Autodesk Fusion 360 part; units mm, degrees
(part 2 of 2)
sketch "Sketch4" plane through (0, 0, 8) normal (0, 0, 1) x (-1, 0, 0)
  line L0 (-123.1754, -6.5) -> (-116.8246, -6.5)
  line L1 (-116.8246, -6.5) -> (-113.6491, -12)
  line L2 (-113.6491, -12) -> (-116.8246, -17.5)
  line L3 (-116.8246, -17.5) -> (-123.1754, -17.5)
  line L4 (-123.1754, -17.5) -> (-126.3509, -12)
  line L5 (-126.3509, -12) -> (-123.1754, -6.5)
  line L6 (-39.1754, -6.5) -> (-32.8246, -6.5)
  line L7 (-32.8246, -6.5) -> (-29.6491, -12)
  line L8 (-29.6491, -12) -> (-32.8246, -17.5)
  line L9 (-32.8246, -17.5) -> (-39.1754, -17.5)
  line L10 (-39.1754, -17.5) -> (-42.3509, -12)
  line L11 (-42.3509, -12) -> (-39.1754, -6.5)
  line L12 (-123.1754, -28.5) -> (-116.8246, -28.5)
  line L13 (-116.8246, -28.5) -> (-113.6491, -34)
  line L14 (-113.6491, -34) -> (-116.8246, -39.5)
  line L15 (-116.8246, -39.5) -> (-123.1754, -39.5)
  line L16 (-123.1754, -39.5) -> (-126.3509, -34)
  line L17 (-126.3509, -34) -> (-123.1754, -28.5)
  line L18 (-39.1754, -28.5) -> (-32.8246, -28.5)
  line L19 (-32.8246, -28.5) -> (-29.6491, -34)
  line L20 (-29.6491, -34) -> (-32.8246, -39.5)
  line L21 (-32.8246, -39.5) -> (-39.1754, -39.5)
  line L22 (-39.1754, -39.5) -> (-42.3509, -34)
  line L23 (-42.3509, -34) -> (-39.1754, -28.5)
  line L24 (-123.1754, -50.5) -> (-116.8246, -50.5)
  line L25 (-116.8246, -50.5) -> (-113.6491, -56)
  line L26 (-113.6491, -56) -> (-116.8246, -61.5)
  line L27 (-116.8246, -61.5) -> (-123.1754, -61.5)
  line L28 (-123.1754, -61.5) -> (-126.3509, -56)
  line L29 (-126.3509, -56) -> (-123.1754, -50.5)
  line L30 (-39.1754, -50.5) -> (-32.8246, -50.5)
  line L31 (-32.8246, -50.5) -> (-29.6491, -56)
  line L32 (-29.6491, -56) -> (-32.8246, -61.5)
  line L33 (-32.8246, -61.5) -> (-39.1754, -61.5)
  line L34 (-39.1754, -61.5) -> (-42.3509, -56)
  line L35 (-42.3509, -56) -> (-39.1754, -50.5)
  line L36 (-123.1754, -72.5) -> (-116.8246, -72.5)
  line L37 (-116.8246, -72.5) -> (-113.6491, -78)
  line L38 (-113.6491, -78) -> (-116.8246, -83.5)
  line L39 (-116.8246, -83.5) -> (-123.1754, -83.5)
  line L40 (-123.1754, -83.5) -> (-126.3509, -78)
  line L41 (-126.3509, -78) -> (-123.1754, -72.5)
  line L42 (-39.1754, -72.5) -> (-32.8246, -72.5)
  line L43 (-32.8246, -72.5) -> (-29.6491, -78)
  line L44 (-29.6491, -78) -> (-32.8246, -83.5)
  line L45 (-32.8246, -83.5) -> (-39.1754, -83.5)
  line L46 (-39.1754, -83.5) -> (-42.3509, -78)
  line L47 (-42.3509, -78) -> (-39.1754, -72.5)
  line L48 (-123.1754, -94.5) -> (-116.8246, -94.5)
  line L49 (-116.8246, -94.5) -> (-113.6491, -100)
  line L50 (-113.6491, -100) -> (-116.8246, -105.5)
  line L51 (-116.8246, -105.5) -> (-123.1754, -105.5)
  line L52 (-123.1754, -105.5) -> (-126.3509, -100)
  line L53 (-126.3509, -100) -> (-123.1754, -94.5)
  line L54 (-39.1754, -94.5) -> (-32.8246, -94.5)
  line L55 (-32.8246, -94.5) -> (-29.6491, -100)
  line L56 (-29.6491, -100) -> (-32.8246, -105.5)
  line L57 (-32.8246, -105.5) -> (-39.1754, -105.5)
  line L58 (-39.1754, -105.5) -> (-42.3509, -100)
  line L59 (-42.3509, -100) -> (-39.1754, -94.5)
  line L60 (-123.1754, -116.5) -> (-116.8246, -116.5)
  line L61 (-116.8246, -116.5) -> (-113.6491, -122)
  line L62 (-113.6491, -122) -> (-116.8246, -127.5)
  line L63 (-116.8246, -127.5) -> (-123.1754, -127.5)
  line L64 (-123.1754, -127.5) -> (-126.3509, -122)
  line L65 (-126.3509, -122) -> (-123.1754, -116.5)
  line L66 (-18.1754, -127.5) -> (-21.3509, -122)
  line L67 (-21.3509, -122) -> (-18.1754, -116.5)
  line L68 (-18.1754, -116.5) -> (-11.8246, -116.5)
  line L69 (-11.8246, -116.5) -> (-8.6491, -122)
  line L70 (-8.6491, -122) -> (-11.8246, -127.5)
  line L71 (-11.8246, -127.5) -> (-18.1754, -127.5)
  line L72 (-60.1754, -116.5) -> (-53.8246, -116.5)
  line L73 (-53.8246, -116.5) -> (-50.6491, -122)
  line L74 (-50.6491, -122) -> (-53.8246, -127.5)
  line L75 (-53.8246, -127.5) -> (-60.1754, -127.5)
  line L76 (-60.1754, -127.5) -> (-63.3509, -122)
  line L77 (-63.3509, -122) -> (-60.1754, -116.5)
  line L78 (-144.1754, -116.5) -> (-137.8246, -116.5)
  line L79 (-137.8246, -116.5) -> (-134.6491, -122)
  line L80 (-134.6491, -122) -> (-137.8246, -127.5)
  line L81 (-137.8246, -127.5) -> (-144.1754, -127.5)
  line L82 (-144.1754, -127.5) -> (-147.3509, -122)
  line L83 (-147.3509, -122) -> (-144.1754, -116.5)
  line L84 (-60.1754, -94.5) -> (-53.8246, -94.5)
  line L85 (-53.8246, -94.5) -> (-50.6491, -100)
  line L86 (-50.6491, -100) -> (-53.8246, -105.5)
  line L87 (-53.8246, -105.5) -> (-60.1754, -105.5)
  line L88 (-60.1754, -105.5) -> (-63.3509, -100)
  line L89 (-63.3509, -100) -> (-60.1754, -94.5)
  line L90 (-144.1754, -94.5) -> (-137.8246, -94.5)
  line L91 (-137.8246, -94.5) -> (-134.6491, -100)
  line L92 (-134.6491, -100) -> (-137.8246, -105.5)
  line L93 (-137.8246, -105.5) -> (-144.1754, -105.5)
  line L94 (-144.1754, -105.5) -> (-147.3509, -100)
  line L95 (-147.3509, -100) -> (-144.1754, -94.5)
  line L96 (-60.1754, -72.5) -> (-53.8246, -72.5)
  line L97 (-53.8246, -72.5) -> (-50.6491, -78)
  line L98 (-50.6491, -78) -> (-53.8246, -83.5)
  line L99 (-53.8246, -83.5) -> (-60.1754, -83.5)
  line L100 (-60.1754, -83.5) -> (-63.3509, -78)
  line L101 (-63.3509, -78) -> (-60.1754, -72.5)
  line L102 (-144.1754, -72.5) -> (-137.8246, -72.5)
  line L103 (-137.8246, -72.5) -> (-134.6491, -78)
  line L104 (-134.6491, -78) -> (-137.8246, -83.5)
  line L105 (-137.8246, -83.5) -> (-144.1754, -83.5)
  line L106 (-144.1754, -83.5) -> (-147.3509, -78)
  line L107 (-147.3509, -78) -> (-144.1754, -72.5)
  line L108 (-60.1754, -50.5) -> (-53.8246, -50.5)
  line L109 (-53.8246, -50.5) -> (-50.6491, -56)
  line L110 (-50.6491, -56) -> (-53.8246, -61.5)
  line L111 (-53.8246, -61.5) -> (-60.1754, -61.5)
  line L112 (-60.1754, -61.5) -> (-63.3509, -56)
  line L113 (-63.3509, -56) -> (-60.1754, -50.5)
  line L114 (-144.1754, -50.5) -> (-137.8246, -50.5)
  line L115 (-137.8246, -50.5) -> (-134.6491, -56)
  line L116 (-134.6491, -56) -> (-137.8246, -61.5)
  line L117 (-137.8246, -61.5) -> (-144.1754, -61.5)
  line L118 (-144.1754, -61.5) -> (-147.3509, -56)
  line L119 (-147.3509, -56) -> (-144.1754, -50.5)
  line L120 (-60.1754, -28.5) -> (-53.8246, -28.5)
  line L121 (-53.8246, -28.5) -> (-50.6491, -34)
  line L122 (-50.6491, -34) -> (-53.8246, -39.5)
  line L123 (-53.8246, -39.5) -> (-60.1754, -39.5)
  line L124 (-60.1754, -39.5) -> (-63.3509, -34)
  line L125 (-63.3509, -34) -> (-60.1754, -28.5)
  line L126 (-144.1754, -28.5) -> (-137.8246, -28.5)
  line L127 (-137.8246, -28.5) -> (-134.6491, -34)
  line L128 (-134.6491, -34) -> (-137.8246, -39.5)
  line L129 (-137.8246, -39.5) -> (-144.1754, -39.5)
  line L130 (-144.1754, -39.5) -> (-147.3509, -34)
  line L131 (-147.3509, -34) -> (-144.1754, -28.5)
  line L132 (-60.1754, -6.5) -> (-53.8246, -6.5)
  line L133 (-53.8246, -6.5) -> (-50.6491, -12)
  line L134 (-50.6491, -12) -> (-53.8246, -17.5)
  line L135 (-53.8246, -17.5) -> (-60.1754, -17.5)
  line L136 (-60.1754, -17.5) -> (-63.3509, -12)
  line L137 (-63.3509, -12) -> (-60.1754, -6.5)
  line L138 (-144.1754, -6.5) -> (-137.8246, -6.5)
  line L139 (-137.8246, -6.5) -> (-134.6491, -12)
  line L140 (-134.6491, -12) -> (-137.8246, -17.5)
  line L141 (-137.8246, -17.5) -> (-144.1754, -17.5)
  line L142 (-144.1754, -17.5) -> (-147.3509, -12)
  line L143 (-147.3509, -12) -> (-144.1754, -6.5)
  line L144 (-102.1754, -6.5) -> (-95.8246, -6.5)
  line L145 (-95.8246, -6.5) -> (-92.6491, -12)
  line L146 (-92.6491, -12) -> (-95.8246, -17.5)
  line L147 (-95.8246, -17.5) -> (-102.1754, -17.5)
  line L148 (-102.1754, -17.5) -> (-105.3509, -12)
  line L149 (-105.3509, -12) -> (-102.1754, -6.5)
  line L150 (-18.1754, -6.5) -> (-11.8246, -6.5)
  line L151 (-11.8246, -6.5) -> (-8.6491, -12)
  line L152 (-8.6491, -12) -> (-11.8246, -17.5)
  line L153 (-11.8246, -17.5) -> (-18.1754, -17.5)
  line L154 (-18.1754, -17.5) -> (-21.3509, -12)
  line L155 (-21.3509, -12) -> (-18.1754, -6.5)
  line L156 (-102.1754, -28.5) -> (-95.8246, -28.5)
  line L157 (-95.8246, -28.5) -> (-92.6491, -34)
  line L158 (-92.6491, -34) -> (-95.8246, -39.5)
  line L159 (-95.8246, -39.5) -> (-102.1754, -39.5)
  line L160 (-102.1754, -39.5) -> (-105.3509, -34)
  line L161 (-105.3509, -34) -> (-102.1754, -28.5)
  line L162 (-18.1754, -28.5) -> (-11.8246, -28.5)
  line L163 (-11.8246, -28.5) -> (-8.6491, -34)
  line L164 (-8.6491, -34) -> (-11.8246, -39.5)
  line L165 (-11.8246, -39.5) -> (-18.1754, -39.5)
  line L166 (-18.1754, -39.5) -> (-21.3509, -34)
  line L167 (-21.3509, -34) -> (-18.1754, -28.5)
  line L168 (-102.1754, -50.5) -> (-95.8246, -50.5)
  line L169 (-95.8246, -50.5) -> (-92.6491, -56)
  line L170 (-92.6491, -56) -> (-95.8246, -61.5)
  line L171 (-95.8246, -61.5) -> (-102.1754, -61.5)
  line L172 (-102.1754, -61.5) -> (-105.3509, -56)
  line L173 (-105.3509, -56) -> (-102.1754, -50.5)
  line L174 (-18.1754, -50.5) -> (-11.8246, -50.5)
  line L175 (-11.8246, -50.5) -> (-8.6491, -56)
  line L176 (-8.6491, -56) -> (-11.8246, -61.5)
  line L177 (-11.8246, -61.5) -> (-18.1754, -61.5)
  line L178 (-18.1754, -61.5) -> (-21.3509, -56)
  line L179 (-21.3509, -56) -> (-18.1754, -50.5)
  line L180 (-102.1754, -72.5) -> (-95.8246, -72.5)
  line L181 (-95.8246, -72.5) -> (-92.6491, -78)
  line L182 (-92.6491, -78) -> (-95.8246, -83.5)
  line L183 (-95.8246, -83.5) -> (-102.1754, -83.5)
  line L184 (-102.1754, -83.5) -> (-105.3509, -78)
  line L185 (-105.3509, -78) -> (-102.1754, -72.5)
  line L186 (-18.1754, -72.5) -> (-11.8246, -72.5)
  line L187 (-11.8246, -72.5) -> (-8.6491, -78)
  line L188 (-8.6491, -78) -> (-11.8246, -83.5)
  line L189 (-11.8246, -83.5) -> (-18.1754, -83.5)
  line L190 (-18.1754, -83.5) -> (-21.3509, -78)
  line L191 (-21.3509, -78) -> (-18.1754, -72.5)
  line L192 (-102.1754, -94.5) -> (-95.8246, -94.5)
  line L193 (-95.8246, -94.5) -> (-92.6491, -100)
  line L194 (-92.6491, -100) -> (-95.8246, -105.5)
  line L195 (-95.8246, -105.5) -> (-102.1754, -105.5)
  line L196 (-102.1754, -105.5) -> (-105.3509, -100)
  line L197 (-105.3509, -100) -> (-102.1754, -94.5)
  line L198 (-18.1754, -94.5) -> (-11.8246, -94.5)
  line L199 (-11.8246, -94.5) -> (-8.6491, -100)
  line L200 (-8.6491, -100) -> (-11.8246, -105.5)
  line L201 (-11.8246, -105.5) -> (-18.1754, -105.5)
  line L202 (-18.1754, -105.5) -> (-21.3509, -100)
  line L203 (-21.3509, -100) -> (-18.1754, -94.5)
  line L204 (-102.1754, -116.5) -> (-95.8246, -116.5)
  line L205 (-95.8246, -116.5) -> (-92.6491, -122)
  line L206 (-92.6491, -122) -> (-95.8246, -127.5)
  line L207 (-95.8246, -127.5) -> (-102.1754, -127.5)
  line L208 (-102.1754, -127.5) -> (-105.3509, -122)
  line L209 (-105.3509, -122) -> (-102.1754, -116.5)
  line L210 (-39.1754, -116.5) -> (-32.8246, -116.5)
  line L211 (-32.8246, -116.5) -> (-29.6491, -122)
  line L212 (-29.6491, -122) -> (-32.8246, -127.5)
  line L213 (-32.8246, -127.5) -> (-39.1754, -127.5)
  line L214 (-39.1754, -127.5) -> (-42.3509, -122)
  line L215 (-42.3509, -122) -> (-39.1754, -116.5)
  line L216 (-81.1754, -116.5) -> (-74.8246, -116.5)
  line L217 (-74.8246, -116.5) -> (-71.6491, -122)
  line L218 (-71.6491, -122) -> (-74.8246, -127.5)
  line L219 (-74.8246, -127.5) -> (-81.1754, -127.5)
  line L220 (-81.1754, -127.5) -> (-84.3509, -122)
  line L221 (-84.3509, -122) -> (-81.1754, -116.5)
  line L222 (-165.1754, -116.5) -> (-158.8246, -116.5)
  line L223 (-158.8246, -116.5) -> (-155.6491, -122)
  line L224 (-155.6491, -122) -> (-158.8246, -127.5)
  line L225 (-158.8246, -127.5) -> (-165.1754, -127.5)
  line L226 (-165.1754, -127.5) -> (-168.3509, -122)
  line L227 (-168.3509, -122) -> (-165.1754, -116.5)
  line L228 (-81.1754, -94.5) -> (-74.8246, -94.5)
  line L229 (-74.8246, -94.5) -> (-71.6491, -100)
  line L230 (-71.6491, -100) -> (-74.8246, -105.5)
  line L231 (-74.8246, -105.5) -> (-81.1754, -105.5)
  line L232 (-81.1754, -105.5) -> (-84.3509, -100)
  line L233 (-84.3509, -100) -> (-81.1754, -94.5)
  line L234 (-165.1754, -94.5) -> (-158.8246, -94.5)
  line L235 (-158.8246, -94.5) -> (-155.6491, -100)
  line L236 (-155.6491, -100) -> (-158.8246, -105.5)
  line L237 (-158.8246, -105.5) -> (-165.1754, -105.5)
  line L238 (-165.1754, -105.5) -> (-168.3509, -100)
  line L239 (-168.3509, -100) -> (-165.1754, -94.5)
  line L240 (-81.1754, -72.5) -> (-74.8246, -72.5)
  line L241 (-74.8246, -72.5) -> (-71.6491, -78)
  line L242 (-71.6491, -78) -> (-74.8246, -83.5)
  line L243 (-74.8246, -83.5) -> (-81.1754, -83.5)
  line L244 (-81.1754, -83.5) -> (-84.3509, -78)
  line L245 (-84.3509, -78) -> (-81.1754, -72.5)
  line L246 (-165.1754, -72.5) -> (-158.8246, -72.5)
  line L247 (-158.8246, -72.5) -> (-155.6491, -78)
  line L248 (-155.6491, -78) -> (-158.8246, -83.5)
  line L249 (-158.8246, -83.5) -> (-165.1754, -83.5)
  line L250 (-165.1754, -83.5) -> (-168.3509, -78)
  line L251 (-168.3509, -78) -> (-165.1754, -72.5)
  line L252 (-81.1754, -50.5) -> (-74.8246, -50.5)
  line L253 (-74.8246, -50.5) -> (-71.6491, -56)
  line L254 (-71.6491, -56) -> (-74.8246, -61.5)
  line L255 (-74.8246, -61.5) -> (-81.1754, -61.5)
  line L256 (-81.1754, -61.5) -> (-84.3509, -56)
  line L257 (-84.3509, -56) -> (-81.1754, -50.5)
  line L258 (-165.1754, -50.5) -> (-158.8246, -50.5)
  line L259 (-158.8246, -50.5) -> (-155.6491, -56)
  line L260 (-155.6491, -56) -> (-158.8246, -61.5)
  line L261 (-158.8246, -61.5) -> (-165.1754, -61.5)
  line L262 (-165.1754, -61.5) -> (-168.3509, -56)
  line L263 (-168.3509, -56) -> (-165.1754, -50.5)
  line L264 (-81.1754, -28.5) -> (-74.8246, -28.5)
  line L265 (-74.8246, -28.5) -> (-71.6491, -34)
  line L266 (-71.6491, -34) -> (-74.8246, -39.5)
  line L267 (-74.8246, -39.5) -> (-81.1754, -39.5)
  line L268 (-81.1754, -39.5) -> (-84.3509, -34)
  line L269 (-84.3509, -34) -> (-81.1754, -28.5)
  line L270 (-165.1754, -28.5) -> (-158.8246, -28.5)
  line L271 (-158.8246, -28.5) -> (-155.6491, -34)
  line L272 (-155.6491, -34) -> (-158.8246, -39.5)
  line L273 (-158.8246, -39.5) -> (-165.1754, -39.5)
  line L274 (-165.1754, -39.5) -> (-168.3509, -34)
  line L275 (-168.3509, -34) -> (-165.1754, -28.5)
  line L276 (-81.1754, -6.5) -> (-74.8246, -6.5)
  line L277 (-74.8246, -6.5) -> (-71.6491, -12)
  line L278 (-71.6491, -12) -> (-74.8246, -17.5)
  line L279 (-74.8246, -17.5) -> (-81.1754, -17.5)
  line L280 (-81.1754, -17.5) -> (-84.3509, -12)
  line L281 (-84.3509, -12) -> (-81.1754, -6.5)
  line L282 (-165.1754, -6.5) -> (-158.8246, -6.5)
  line L283 (-158.8246, -6.5) -> (-155.6491, -12)
  line L284 (-155.6491, -12) -> (-158.8246, -17.5)
  line L285 (-158.8246, -17.5) -> (-165.1754, -17.5)
  line L286 (-165.1754, -17.5) -> (-168.3509, -12)
  line L287 (-168.3509, -12) -> (-165.1754, -6.5)
  line L288 (0, -132) -> (0, 0)
  line L289 (0, 0) -> (-176, 0)
  line L290 (-176, 0) -> (-176, -132)
  line L291 (-176, -132) -> (0, -132)
  circle A0 centre (-15, -122) radius 2.875
  line L292 (-176, -12) -> (0, -12) construction
  line L293 (-176, -34) -> (0, -34) construction
  line L294 (-176, -56) -> (0, -56) construction
  line L295 (-176, -78) -> (0, -78) construction
  line L296 (-176, -100) -> (0, -100) construction
  line L297 (-176, -122) -> (0, -122) construction
  line L298 (-162, -6.5) -> (-162, 0) construction
  line L299 (-141, -6.5) -> (-141, 0) construction
  line L300 (-120, -6.5) -> (-120, 0) construction
  line L301 (-99, -6.5) -> (-99, 0) construction
  line L302 (-78, -6.5) -> (-78, 0) construction
  line L303 (-57, -6.5) -> (-57, 0) construction
  line L304 (-36, -6.5) -> (-36, 0) construction
  line L305 (-15, -6.5) -> (-15, 0) construction
  line L306 (-162, -6.5) -> (-162, -132) construction
  line L307 (-141, -6.5) -> (-141, -132) construction
  line L308 (-120, -6.5) -> (-120, -132) construction
  line L309 (-99, -6.5) -> (-99, -132) construction
  line L310 (-78, -6.5) -> (-78, -132) construction
  line L311 (-57, -6.5) -> (-57, -132) construction
  line L312 (-36, -6.5) -> (-36, -132) construction
  line L313 (-15, -6.5) -> (-15, -132) construction
  circle A1 centre (-162, -12) radius 2.875
  circle A2 centre (-141, -12) radius 2.875
  circle A3 centre (-120, -12) radius 2.875
  circle A4 centre (-99, -12) radius 2.875
  circle A5 centre (-78, -12) radius 2.875
  circle A6 centre (-57, -12) radius 2.875
  circle A7 centre (-36, -12) radius 2.875
  circle A8 centre (-15, -12) radius 2.875
  circle A9 centre (-162, -34) radius 2.875
  circle A10 centre (-141, -34) radius 2.875
  circle A11 centre (-120, -34) radius 2.875
  circle A12 centre (-99, -34) radius 2.875
  circle A13 centre (-78, -34) radius 2.875
  circle A14 centre (-57, -34) radius 2.875
  circle A15 centre (-36, -34) radius 2.875
  circle A16 centre (-15, -34) radius 2.875
  circle A17 centre (-162, -56) radius 2.875
  circle A18 centre (-141, -56) radius 2.875
  circle A19 centre (-120, -56) radius 2.875
  circle A20 centre (-99, -56) radius 2.875
  circle A21 centre (-78, -56) radius 2.875
  circle A22 centre (-57, -56) radius 2.875
  circle A23 centre (-36, -56) radius 2.875
  circle A24 centre (-15, -56) radius 2.875
  circle A25 centre (-162, -78) radius 2.875
  circle A26 centre (-141, -78) radius 2.875
  circle A27 centre (-120, -78) radius 2.875
  circle A28 centre (-99, -78) radius 2.875
  circle A29 centre (-78, -78) radius 2.875
  circle A30 centre (-57, -78) radius 2.875
  circle A31 centre (-36, -78) radius 2.875
  circle A32 centre (-15, -78) radius 2.875
  circle A33 centre (-162, -100) radius 2.875
  circle A34 centre (-141, -100) radius 2.875
  circle A35 centre (-120, -100) radius 2.875
  circle A36 centre (-99, -100) radius 2.875
  circle A37 centre (-78, -100) radius 2.875
  circle A38 centre (-57, -100) radius 2.875
  circle A39 centre (-36, -100) radius 2.875
  circle A40 centre (-15, -100) radius 2.875
  circle A41 centre (-162, -122) radius 2.875
  circle A42 centre (-141, -122) radius 2.875
  circle A43 centre (-120, -122) radius 2.875
  circle A44 centre (-99, -122) radius 2.875
  circle A45 centre (-78, -122) radius 2.875
  circle A46 centre (-57, -122) radius 2.875
  circle A47 centre (-36, -122) radius 2.875
  dimension "d18" = 12
  constraint coincident L288 L292.end
  constraint perpendicular L288 L292
  constraint coincident L290 L293.start
  constraint coincident L288 L293.end
  constraint perpendicular L288 L293
  constraint coincident L290 L294.start
  constraint coincident L288 L294.end
  constraint perpendicular L288 L294
  constraint coincident L290 L295.start
  constraint coincident L288 L295.end
  constraint perpendicular L288 L295
  constraint coincident L290 L296.start
  constraint coincident L288 L296.end
  constraint perpendicular L288 L296
  constraint coincident L290 L297.start
  constraint coincident L288 L297.end
  constraint perpendicular L288 L297
  constraint coincident L274.end L293
  constraint coincident L262.end L294
  constraint coincident L250.end L295
  constraint coincident L238.end L296
  constraint coincident L226.end L297
  constraint midpoint L282 L298.start
  constraint coincident L289 L298.end
  constraint perpendicular L289 L298
  constraint midpoint L138 L299.start
  constraint coincident L289 L299.end
  constraint perpendicular L289 L299
  constraint midpoint L0 L300.start
  constraint coincident L289 L300.end
  constraint perpendicular L289 L300
  constraint midpoint L144 L301.start
  constraint coincident L289 L301.end
  constraint perpendicular L289 L301
  constraint midpoint L276 L302.start
  constraint coincident L289 L302.end
  constraint perpendicular L289 L302
  constraint midpoint L132 L303.start
  constraint coincident L289 L303.end
  constraint perpendicular L289 L303
  constraint midpoint L6 L304.start
  constraint coincident L289 L304.end
  constraint perpendicular L289 L304
  constraint midpoint L150 L305.start
  constraint coincident L289 L305.end
  constraint perpendicular L289 L305
  constraint coincident L291 L306.end
  constraint perpendicular L291 L306
  constraint coincident L291 L307.end
  constraint perpendicular L291 L307
  constraint coincident L291 L308.end
  constraint perpendicular L291 L308
  constraint coincident L291 L309.end
  constraint perpendicular L291 L309
  constraint coincident L291 L310.end
  constraint perpendicular L291 L310
  constraint coincident L291 L311.end
  constraint perpendicular L291 L311
  constraint coincident L291 L312.end
  constraint perpendicular L291 L312
  constraint coincident L291 L313.end
  constraint perpendicular L291 L313
  constraint coincident L292 A1.centre
  constraint coincident L306 A1.centre
  constraint coincident L307 A2.centre
  constraint coincident L292 A2.centre
  constraint coincident L308 A3.centre
  constraint coincident L292 A3.centre
  constraint coincident L292 A4.centre
  constraint coincident L309 A4.centre
  constraint coincident L292 A5.centre
  constraint coincident L310 A5.centre
  constraint coincident L311 A6.centre
  constraint coincident L292 A6.centre
  constraint coincident L312 A7.centre
  constraint coincident L292 A7.centre
  constraint coincident L313 A8.centre
  constraint coincident L292 A8.centre
  constraint coincident L306 A9.centre
  constraint coincident L293 A9.centre
  constraint coincident L307 A10.centre
  constraint coincident L293 A10.centre
  constraint coincident L308 A11.centre
  constraint coincident L293 A11.centre
  constraint coincident L293 A12.centre
  constraint coincident L309 A12.centre
  constraint coincident L293 A13.centre
  constraint coincident L310 A13.centre
  constraint coincident L311 A14.centre
  constraint coincident L293 A14.centre
  constraint coincident L293 A15.centre
  constraint coincident L312 A15.centre
  constraint coincident L313 A16.centre
  constraint coincident L293 A16.centre
  constraint coincident L306 A17.centre
  constraint coincident L294 A17.centre
  constraint coincident L307 A18.centre
  constraint coincident L294 A18.centre
  constraint coincident L294 A19.centre
  constraint coincident L308 A19.centre
  constraint coincident L309 A20.centre
  constraint coincident L294 A20.centre
  constraint coincident L310 A21.centre
  constraint coincident L294 A21.centre
  constraint coincident L311 A22.centre
  constraint coincident L294 A22.centre
  constraint coincident L312 A23.centre
  constraint coincident L294 A23.centre
  constraint coincident L313 A24.centre
  constraint coincident L294 A24.centre
  constraint coincident L295 A25.centre
  constraint coincident L306 A25.centre
  constraint coincident L295 A26.centre
  constraint coincident L307 A26.centre
  constraint coincident L308 A27.centre
  constraint coincident L295 A27.centre
  constraint coincident L295 A28.centre
  constraint coincident L309 A28.centre
  constraint coincident L310 A29.centre
  constraint coincident L295 A29.centre
  constraint coincident L295 A30.centre
  constraint coincident L311 A30.centre
  constraint coincident L312 A31.centre
  constraint coincident L295 A31.centre
  constraint coincident L313 A32.centre
  constraint coincident L295 A32.centre
  constraint coincident L296 A33.centre
  constraint coincident L306 A33.centre
  constraint coincident L307 A34.centre
  constraint coincident L296 A34.centre
  constraint coincident L308 A35.centre
  constraint coincident L296 A35.centre
  constraint coincident L309 A36.centre
  constraint coincident L296 A36.centre
  constraint coincident L310 A37.centre
  constraint coincident L296 A37.centre
  constraint coincident L311 A38.centre
  constraint coincident L296 A38.centre
  constraint coincident L312 A39.centre
  constraint coincident L296 A39.centre
  constraint coincident L313 A40.centre
  constraint coincident L296 A40.centre
  constraint coincident L306 A41.centre
  constraint coincident L297 A41.centre
  constraint coincident L307 A42.centre
  constraint coincident L297 A42.centre
  constraint coincident L308 A43.centre
  constraint coincident L297 A43.centre
  constraint coincident L309 A44.centre
  constraint coincident L297 A44.centre
  constraint coincident L310 A45.centre
  constraint coincident L297 A45.centre
  constraint coincident L297 A46.centre
  constraint coincident L311 A46.centre
  constraint coincident L312 A47.centre
  constraint coincident L297 A47.centre
  constraint equal A41 A42
  constraint equal A42 A43
  constraint equal A43 A44
  constraint equal A44 A45
  constraint equal A45 A46
  constraint equal A46 A47
  constraint equal A39 A47
  constraint equal A38 A39
  constraint equal A37 A38
  constraint equal A36 A37
  constraint equal A35 A36
  constraint equal A34 A35
  constraint equal A33 A34
  constraint equal A33 A40
  constraint equal A25 A40
  constraint equal A25 A26
  constraint equal A26 A27
  constraint equal A27 A28
  constraint equal A28 A29
  constraint equal A29 A30
  constraint equal A30 A31
  constraint equal A31 A32
  constraint equal A24 A32
  constraint equal A23 A24
  constraint equal A22 A23
  constraint equal A21 A22
  constraint equal A20 A21
  constraint equal A19 A20
  constraint equal A18 A19
  constraint equal A17 A18
  constraint equal A9 A17
  constraint equal A9 A10
  constraint equal A10 A11
  constraint equal A11 A12
  constraint equal A12 A13
  constraint equal A13 A14
  constraint equal A14 A15
  constraint equal A15 A16
  constraint equal A0 A16
  constraint equal A1 A2
  constraint equal A2 A3
  constraint equal A3 A4
  constraint equal A4 A5
  constraint equal A5 A6
  constraint equal A6 A7
  constraint equal A7 A8
  constraint equal A8 A9
  measures "d18" distance of L289 L292
extrude "Extrude4" cut sketch "Sketch4" against normal up to surface (8 mm away) contours A1 | A2 | A3 | A4 | A5 | A6 | A7 | A8 | A9 | A10 | A11 | A12 | A13 | A14 | A15 | A16 | A17 | A18 | A19 | A20 | A21 | A22 | A23 | A24 | A25 | A26 | A27 | A28 | A29 | A30 | A31 | A32 | A33 | A34 | A35 | A36 | A37 | A38 | A39 | A40 | A41 | A42 | A43 | A44 | A45 | A46 | A47
equation "d1 = ( 22 * 6 ) * 1 mm"
equation "d2 = ( 8 * 22 ) * 1 mm"
